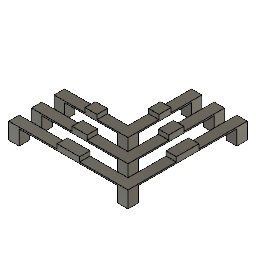
bear_bridge_35-50-65 (Autodesk Fusion 360 design; units mm, degrees)
Autodesk Fusion 360 part; units mm, degrees
sketch "Sketch1" plane through (0, 0, 0) normal (0, 0, 1) x (1, 0, 0)
  line L0 (0, 0) -> (-72, 0)
  line L1 (-72, 0) -> (-72, 7)
  line L2 (-72, 7) -> (7, 7)
  line L3 (0, 0) -> (7, 0)
  line L4 (7, 0) -> (7, 79)
  line L5 (7, 79) -> (0, 79)
  line L6 (0, 79) -> (0, 0)
  line L7 (-65, 7) -> (-65, 0)
  line L8 (0, 72) -> (7, 72)
  line L9 (-40, 7) -> (-40, 0)
  line L10 (-25, 7) -> (-25, 0)
  line L11 (0, 47) -> (7, 47)
  line L12 (0, 32) -> (7, 32)
  line L13 (-32.5, 7) -> (-32.5, 0) construction
  line L14 (0, 39.5) -> (7, 39.5) construction
  line L15 (-72, 22) -> (-8, 22)
  line L16 (-15, 15) -> (-72, 15)
  line L17 (-72, 15) -> (-72, 22)
  line L18 (-15, 15) -> (-8, 15)
  line L19 (-8, 15) -> (-8, 79)
  line L20 (-8, 79) -> (-15, 79)
  line L21 (-15, 79) -> (-15, 15)
  line L22 (-65, 22) -> (-65, 15)
  line L23 (-15, 72) -> (-8, 72)
  line L24 (-45, 22) -> (-45, 15)
  line L25 (-35, 22) -> (-35, 15)
  line L26 (-40, 22) -> (-40, 15) construction
  line L27 (-15, 42) -> (-8, 42)
  line L28 (-15, 52) -> (-8, 52)
  line L29 (-15, 47) -> (-8, 47) construction
  line L30 (-72, 37) -> (-23, 37)
  line L31 (-30, 30) -> (-72, 30)
  line L32 (-72, 30) -> (-72, 37)
  line L33 (-30, 30) -> (-23, 30)
  line L34 (-23, 30) -> (-23, 79)
  line L35 (-23, 79) -> (-30, 79)
  line L36 (-30, 79) -> (-30, 30)
  line L37 (-30, 72) -> (-23, 72)
  line L38 (-65, 30) -> (-65, 37)
  line L39 (-51.5, 37) -> (-51.5, 30)
  line L40 (-43.5, 37) -> (-43.5, 30)
  line L41 (-30, 58.5) -> (-23, 58.5)
  line L42 (-30, 50.5) -> (-23, 50.5)
  line L43 (-47.5, 37) -> (-47.5, 30) construction
  line L44 (-23, 54.5) -> (-30, 54.5) construction
  dimension "d1" = 7
  dimension "d2" = 7
  dimension "d3" = 7
  dimension "d4" = 7
  dimension "d6" = 65
  dimension "d7" = 65
  dimension "d10" = 15
  dimension "d11" = 15
  dimension "d17" = 7
  dimension "d18" = 7
  dimension "d19" = 50
  dimension "d20" = 50
  dimension "d21" = 10
  dimension "d22" = 10
  dimension "d23" = 7
  dimension "d24" = 7
  dimension "d25" = 35
  dimension "d26" = 35
  dimension "d27" = 8
  dimension "d28" = 8
  constraint horizontal L0
  constraint vertical L1
  constraint horizontal L2
  constraint coincident L0.start L3.start
  constraint horizontal L3
  constraint vertical L4
  constraint horizontal L5
  constraint vertical L6
  constraint coincident L2.end L4
  constraint coincident L2 L7.start
  constraint coincident L0 L7.end
  constraint perpendicular L0 L7
  constraint coincident L6 L8.start
  constraint coincident L4 L8.end
  constraint perpendicular L4 L8
  constraint coincident L2 L9.start
  constraint coincident L0 L9.end
  constraint perpendicular L0 L9
  constraint coincident L2 L10.start
  constraint coincident L0 L10.end
  constraint perpendicular L0 L10
  constraint coincident L6 L11.start
  constraint coincident L4 L11.end
  constraint perpendicular L4 L11
  constraint coincident L6 L12.start
  constraint coincident L4 L12.end
  constraint perpendicular L4 L12
  constraint coincident L2 L13.start
  constraint coincident L0 L13.end
  constraint perpendicular L0 L13
  constraint midpoint L2 L13.start
  constraint symmetric L9 L10 L13
  constraint coincident L6 L14.start
  constraint coincident L4 L14.end
  constraint perpendicular L4 L14
  constraint midpoint L4 L14.end
  constraint symmetric L11 L12 L14
  constraint horizontal L15
  constraint horizontal L16
  constraint vertical L17
  constraint horizontal L18
  constraint vertical L19
  constraint horizontal L20
  constraint vertical L21
  constraint coincident L15.end L19
  constraint coincident L15 L22.start
  constraint coincident L16 L22.end
  constraint perpendicular L16 L22
  constraint coincident L21 L23.start
  constraint coincident L19 L23.end
  constraint perpendicular L19 L23
  constraint collinear L5 L20
  constraint collinear L8 L23
  constraint collinear L7 L22
  constraint collinear L1 L17
  constraint coincident L15 L24.start
  constraint coincident L16 L24.end
  constraint perpendicular L16 L24
  constraint coincident L15 L25.start
  constraint coincident L16 L25.end
  constraint perpendicular L16 L25
  constraint midpoint L15 L26.start
  constraint coincident L16 L26.end
  constraint perpendicular L16 L26
  constraint coincident L21 L27.start
  constraint coincident L19 L27.end
  constraint perpendicular L19 L27
  constraint coincident L21 L28.start
  constraint coincident L19 L28.end
  constraint perpendicular L19 L28
  constraint midpoint L21 L29.start
  constraint midpoint L19 L29.end
  constraint symmetric L27 L28 L29
  constraint symmetric L24 L25 L26
  constraint horizontal L30
  constraint horizontal L31
  constraint vertical L32
  constraint horizontal L33
  constraint vertical L34
  constraint horizontal L35
  constraint vertical L36
  constraint coincident L36 L37.start
  constraint coincident L34 L37.end
  constraint perpendicular L34 L37
  constraint coincident L31 L38.start
  constraint coincident L30 L38.end
  constraint perpendicular L30 L38
  constraint coincident L30 L39.start
  constraint coincident L31 L39.end
  constraint perpendicular L31 L39
  constraint coincident L30 L40.start
  constraint coincident L31 L40.end
  constraint perpendicular L31 L40
  constraint coincident L36 L41.start
  constraint coincident L34 L41.end
  constraint perpendicular L34 L41
  constraint coincident L36 L42.start
  constraint coincident L34 L42.end
  constraint perpendicular L34 L42
  constraint coincident L30.end L34
  constraint collinear L17 L32
  constraint collinear L22 L38
  constraint collinear L23 L37
  constraint collinear L20 L35
  constraint midpoint L30 L43.start
  constraint coincident L31 L43.end
  constraint perpendicular L31 L43
  constraint midpoint L34 L44.start
  constraint midpoint L36 L44.end
  constraint symmetric L41 L42 L44
  constraint symmetric L39 L40 L43
  measures "d1" distance of L0.end L1.end
  measures "d2" distance of L0.start L3.end
  measures "d3" distance of L1 L7
  measures "d4" distance of L5 L8
  measures "d6" distance of L6 L7
  measures "d7" distance of L2 L8
  measures "d10" distance of L9 L10
  measures "d11" distance of L11 L12
  measures "d17" distance of L19.end L20.end
  measures "d18" distance of L15.start L16.end
  measures "d19" distance of L21 L22
  measures "d20" distance of L15 L23
  measures "d21" distance of L24 L25
  measures "d22" distance of L27 L28
  measures "d23" distance of L34 L36 L0.end
  measures "d24" distance of L30 L33
  measures "d25" distance of L36 L38
  measures "d26" distance of L30 L37
  measures "d27" distance of L39 L40
  measures "d28" distance of L41 L42
extrude "Extrude1" add sketch "Sketch1" against normal blind 10 contours L2 L3 L4 L6 | L0 L1 L2 L7 | L4 L5 L6 L8 | L15 L16 L17 L22 | L15 L18 L19 L21 | L19 L20 L21 L23 | L30 L31 L32 L38 | L30 L33 L34 L36 | L34 L35 L36 L37 makes body 1 at (-72, 2.3333, -3.3333) makes body 2 at (7, 2.3333, -3.3333) makes body 3 at (4.6667, 79, -3.3333) makes body 4 at (-23, 32.3333, -3.3333) makes body 5 at (-8, 17.3333, -3.3333) makes body 6 at (-30, 76.6667, -6.6667) makes body 7 at (-65, 19.6667, -3.3333) makes body 8 at (-69.6667, 37, -6.6667) makes body 9 at (-10.3333, 79, -3.3333)
extrude "Extrude2" add sketch "Sketch1" along normal blind 1 bodies 4 5 2 6 7 8 9 1 3
extrude "Extrude3" add sketch "Sketch1" along normal blind 3 from surface at 1 contours L0 L2 L9 L10 | L4 L6 L11 L12 | L15 L16 L24 L25 | L19 L21 L27 L28 | L30 L31 L39 L40 | L34 L36 L41 L42 bodies 4 5 2
equation "d1 = d2"
equation "d3 = d2"
equation "d4 = d2"
equation "d7 = d6"
equation "d11 = d10"
equation "d17 = d2"
equation "d18 = d2"
equation "d19 = d6 - 15 mm"
equation "d20 = d6 - 15 mm"
equation "d22 = d21"
equation "d23 = d2"
equation "d24 = d2"
equation "d25 = d19 - 15 mm"
equation "d26 = d19 - 15 mm"
equation "d28 = d27"
